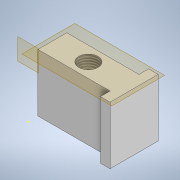
# Autodesk Inventor part: SoporteHerramienta
Saved by Autodesk Inventor 2020 (Build 240168000, 168)
## iProperties
Created: 2019-09-28
Part Number: SoporteHerramienta
Material: Genérico
Document SubType Name: Modeling
Designer: Java9
Density: 1 g/cm^3
Appearance: Valor por defecto
Author: Java9
Autodesk Inventor part; units mm, degrees
ref_plane "YZ Plane" through (0, 0, 0) normal (1, 0, 0) x (0, 1, 0)
ref_plane "XZ Plane" through (0, 0, 0) normal (0, 1, 0) x (-1, 0, 0)
ref_plane "XY Plane" through (0, 0, 0) normal (0, 0, 1) x (1, 0, 0)
sketch "Boceto1" plane through (0, 0, 0) normal (0, 0, 1) x (1, 0, 0)
  line L0 (0, 0) -> (85, 0)
  line L1 (85, 0) -> (85, 60)
  line L2 (0, 60) -> (0, 0)
  line L3 (0, 60) -> (85, 60)
  dimension "d0" = 85
  dimension "d1" = 60
  constraints: 8 end point, 2 horizontal, 1 parallel, 1 perpendicular
  measures "d0" distance of L2.start L1.end
  measures "d1" distance of L1.end L0.end
extrude "Extrusión1" add sketch "Boceto1" along normal blind 50
sketch "Boceto3" plane through (0, 0, 50) normal (0, 0, 1) x (1, 0, 0)
  point P0 (0, 0)
ref_plane "Plano de trabajo3" through (0, 60, 50) normal (0, 0, 1) x (1, 0, 0)
sketch "Boceto4" plane through (0, 60, 50) normal (0, 0, 1) x (1, 0, 0)
  line L0 (0, -60) -> (85, -60) projected
  line L1 (0, -60) -> (75, -60)
  line L2 (75, -60) -> (75, 0)
  line L3 (75, 0) -> (0, 0)
  line L4 (0, 0) -> (0, -60) projected
  line L5 (0, 0) -> (0, -60)
  dimension "d7" = 75
  dimension "d8" = 60
  constraints: 8 end point, 2 perpendicular, 1 collinear, 1 point on line
  measures "d7" distance of L0.start L1.end
  measures "d8" distance of L1.end L2.end
extrude "Extrusión2" cut sketch "Boceto4" against normal blind 10
sketch "Boceto5" plane through (0, 0, 0) normal (0, 0, -1) x (-1, 0, 0)
  line L0 (0, 0) -> (-85, 0) projected
  line L1 (0, 0) -> (-75, 0)
  line L2 (-75, 0) -> (-75, 60)
  line L3 (-85, 60) -> (0, 60) projected
  line L4 (-75, 60) -> (0, 60)
  line L5 (0, 60) -> (0, 0) projected
  line L6 (0, 60) -> (0, 0)
  dimension "d11" = 75
  dimension "d12" = 60
  constraints: 8 end point, 1 perpendicular, 1 point on line
  measures "d11" distance of L0.start L1.end
  measures "d12" distance of L1.end L2.end
extrude "Extrusión3" cut sketch "Boceto5" against normal blind 10
ref_plane "Plano de trabajo5" through (85, 60, 50) normal (0, 1, 0) x (1, 0, 0)
sketch "Boceto6" plane through (85, 60, 50) normal (0, 1, 0) x (1, 0, 0)
  line L0 (-85, 10) -> (-10, 10) projected
  line L1 (-10, 40) -> (-85, 40) projected
  circle A0 centre (-47.5, 25) radius 10
  point P0 (-85, 50)
  dimension "d15" = 20
  constraints: 1 centre point
  measures "d15" diameter of A0
extrude "Extrusión4" cut sketch "Boceto6" against normal through all
thread "Rosca1" size "M20x2.5" class "6H" standard "ANSI Metric M Profile" full length
